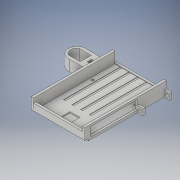
# Autodesk Inventor part: PI_Box_FINAL_COPY2
Saved by Autodesk Inventor 2017 (Build 210142000, 142)
## iProperties
Created: 2020-02-08
Part Number: PI_Box_FINAL_COPY2
Material: Generic
Document SubType Name: Modeling
Designer: S346559073
Density: 1 g/cm^3
Appearance: Default
Author: S346559073
Autodesk Inventor part; units mm, degrees
ref_plane "YZ Plane" through (0, 0, 0) normal (1, 0, 0) x (0, 1, 0)
ref_plane "XZ Plane" through (0, 0, 0) normal (0, 1, 0) x (-1, 0, 0)
ref_plane "XY Plane" through (0, 0, 0) normal (0, 0, 1) x (1, 0, 0)
sketch "Sketch1" plane through (0, 0, 0) normal (0, 1, 0) x (-1, 0, 0)
  line L0 (0, 0) -> (55.88, 0)
  line L1 (55.88, 0) -> (55.88, 88.9)
  line L2 (55.88, 88.9) -> (0, 88.9)
  line L3 (0, 88.9) -> (0, 0)
  dimension "d0" = 55.88
  dimension "d1" = 88.9
  constraints: 8 end point, 2 parallel, 1 horizontal, 1 perpendicular
  measures "d0" distance of L2.end L1.end
  measures "d1" distance of L0.end L1.end
extrude "Extrusion1" add sketch "Sketch1" along normal blind 2.54
sketch "Sketch2" plane through (0, 2.54, 0) normal (0, 1, 0) x (1, 0, 0)
  line L0 (-55.88, -88.9) -> (0, -88.9) projected
  line L1 (-22.86, -88.9) -> (-34.29, -88.9)
  line L2 (-34.29, -88.9) -> (-34.29, -72.771)
  line L3 (-34.29, -72.771) -> (-22.86, -72.771)
  line L4 (-22.86, -72.771) -> (-22.86, -88.9)
  point P0 (0, 0)
  dimension "d4" = 11.43
  dimension "d5" = 16.129
  dimension "d6" = 21.59
  dimension "d7" = 22.86
  constraints: 8 end point, 2 parallel, 1 horizontal, 1 perpendicular, 1 point on line
  measures "d4" distance of L2.end L3.end
  measures "d5" distance of L1.end L2.end
  measures "d6" distance of L0.start L1.end
  measures "d7" distance of L0.end L1.start
extrude "Extrusion2" cut sketch "Sketch2" against normal blind 1.27
sketch "Sketch3" plane through (0, 2.54, 0) normal (0, 1, 0) x (1, 0, 0)
  line L0 (-10.5239, -64.7488) -> (-8.3034, -64.7488)
  line L1 (-8.3034, -64.7488) -> (-8.3034, 0)
  line L2 (-8.3034, 0) -> (-10.5239, 0)
  line L3 (-10.5239, 0) -> (-10.5239, -64.7488)
  line L4 (0, 0) -> (-55.88, 0) projected
  line L5 (-27.9843, -64.7488) -> (-30.2048, -64.7488)
  line L6 (-30.2048, -64.7488) -> (-30.2048, 0)
  line L7 (-30.2048, 0) -> (-27.9843, 0)
  line L8 (-27.9843, 0) -> (-27.9843, -64.7488)
  line L9 (-49.8857, -64.7488) -> (-47.6652, -64.7488)
  line L10 (-47.6652, -64.7488) -> (-47.6652, 0)
  line L11 (-47.6652, 0) -> (-49.8857, 0)
  line L12 (-49.8857, 0) -> (-49.8857, -64.7488)
  line L13 (-40.0452, -64.7488) -> (-37.8248, -64.7488)
  line L14 (-37.8248, -64.7488) -> (-37.8248, 0)
  line L15 (-37.8248, 0) -> (-40.0452, 0)
  line L16 (-40.0452, 0) -> (-40.0452, -64.7488)
  line L17 (-20.3643, -64.7488) -> (-18.1439, -64.7488)
  line L18 (-18.1439, -64.7488) -> (-18.1439, 0)
  line L19 (-18.1439, 0) -> (-20.3643, 0)
  line L20 (-20.3643, 0) -> (-20.3643, -64.7488)
  line L21 (-47.6652, -64.7488) -> (-40.0452, -64.7488)
  line L22 (-34.29, -72.771) -> (-22.86, -72.771) projected
  line L23 (-37.8248, -64.7488) -> (-30.2048, -64.7488)
  line L24 (-27.9843, -64.7488) -> (-20.3643, -64.7488)
  line L25 (-18.1439, -64.7488) -> (-10.5239, -64.7488)
  dimension "d10" = 7.62
  constraints: 48 end point, 11 parallel, 9 collinear, 8 point on line, 6 perpendicular, 5 horizontal
  measures "d10" distance of L5.start L17.start
extrude "Extrusion3" cut sketch "Sketch3" against normal blind 0.508 contours L3 L2 L1 L0 | L17 L20 L4 L18 | L5 L6 L4 L8 | L13 L16 L4 L14 | L9 L12 L4 L10
sketch "Sketch4" plane through (-55.88, 0, 0) normal (-1, 0, 0) x (0, 0, 1)
  line L0 (88.9, 0) -> (0, 0) projected
  line L1 (88.9, 0) -> (0, 0)
  line L2 (0, 0) -> (0, 2.54)
  line L3 (0, 2.54) -> (88.9, 2.54)
  line L4 (88.9, 2.54) -> (88.9, 0)
  constraints: 8 end point, 2 parallel, 1 horizontal, 1 perpendicular
extrude "Extrusion4" add sketch "Sketch4" along normal blind 2.54
sketch "Sketch5" plane through (0, 2.54, 0) normal (0, 1, 0) x (1, 0, 0)
  line L0 (0, -88.9) -> (-58.42, -88.9) projected
  line L1 (-49.8857, 0) -> (-58.42, 0) projected
  line L2 (-58.42, -88.9) -> (-55.88, -88.9)
  line L3 (-55.88, -88.9) -> (-55.88, 0)
  line L4 (-55.88, 0) -> (-58.42, 0)
  line L5 (-58.42, 0) -> (-58.42, -88.9)
  point P0 (0, 0)
  dimension "d15" = 2.54
  constraints: 8 end point, 2 parallel, 1 horizontal, 1 perpendicular, 1 point on line
  measures "d15" distance of L4.end L3.end
extrude "Extrusion5" add sketch "Sketch5" along normal blind 12.7
sketch "Sketch6" plane through (0, 0, 88.9) normal (1, 0, 0) x (0, 0, -1)
  line L0 (0, 2.54) -> (16.129, 2.54) projected
  line L1 (0, 0) -> (88.9, 0) projected
  line L2 (0, 2.54) -> (88.9, 2.54)
  line L3 (88.9, 2.54) -> (88.9, 0)
  line L4 (88.9, 0) -> (0, 0)
  line L5 (0, 0) -> (0, 2.54)
  constraints: 8 end point, 2 parallel, 1 horizontal, 1 perpendicular
extrude "Extrusion6" add sketch "Sketch6" along normal blind 2.54
sketch "Sketch7" plane through (0, 2.54, 0) normal (0, 1, 0) x (1, 0, 0)
  line L0 (2.54, 0) -> (2.54, -88.9) projected
  line L1 (2.54, -88.9) -> (0, -88.9)
  line L2 (0, -88.9) -> (0, 0)
  line L3 (0, 0) -> (2.54, 0)
  line L4 (2.54, 0) -> (2.54, -88.9)
  constraints: 8 end point, 2 parallel, 1 horizontal, 1 perpendicular
extrude "Extrusion7" add sketch "Sketch7" along normal blind 12.7
sketch "Sketch8" plane through (-34.29, 1.27, 88.9) normal (0, 0, 1) x (1, 0, 0)
  line L0 (-24.13, -1.27) -> (-24.13, 13.97) projected
  line L1 (-21.59, 1.27) -> (-21.59, 13.97) projected
  line L2 (-24.13, 13.97) -> (-21.59, 13.97)
  line L3 (-21.59, 13.97) -> (-21.59, 1.27)
  line L4 (-21.59, 1.27) -> (-24.13, 1.27)
  line L5 (-24.13, 1.27) -> (-24.13, 13.97)
  line L6 (-24.13, 1.27) -> (36.83, 1.27)
  line L7 (36.83, 1.27) -> (36.83, 3.0441)
  line L8 (36.83, 3.0441) -> (-24.13, 3.0441)
  line L9 (-24.13, 3.0441) -> (-24.13, 1.27)
  line L10 (36.83, -1.27) -> (36.83, 13.97) projected
  line L11 (34.29, 1.27) -> (36.83, 1.27)
  line L12 (36.83, 1.27) -> (36.83, 13.97)
  line L13 (36.83, 13.97) -> (34.29, 13.97)
  line L14 (34.29, 13.97) -> (34.29, 1.27)
  line L15 (13.9257, 1.27) -> (6.3057, 1.27) projected
  line L16 (11.43, 0) -> (0, 0) projected
  line L17 (11.3074, 1.27) -> (0, 1.27)
  line L18 (0, 1.27) -> (0, 0)
  line L19 (0, 0) -> (11.3074, 0)
  line L20 (11.3074, 0) -> (11.3074, 1.27)
  point P0 (34.29, -1.27)
  constraints: 32 end point, 8 parallel, 4 horizontal, 4 perpendicular, 2 point on line
extrude "Extrusion8" add sketch "Sketch8" along normal blind 3.81 contours L0 L8 L1 L4 | L0 L2 L1 L8 | L1 L8 L14 L6 | L14 L13 L10 L8 | L8 L7 L6 L14
sketch "Sketch9" plane through (0, 2.54, 0) normal (0, 1, 0) x (1, 0, 0)
  line L0 (0, -92.71) -> (-55.88, -92.71) projected
  line L1 (-55.8607, -92.71) -> (0, -92.71)
  line L2 (0, -92.71) -> (0, -90.17)
  line L3 (0, -90.17) -> (-55.8607, -90.17)
  line L4 (-55.8607, -90.17) -> (-55.8607, -92.71)
  point P0 (0, 0)
  point P1 (-58.42, -92.71)
  point P2 (2.54, -92.71)
  dimension "d24" = 2.54
  constraints: 8 end point, 2 parallel, 1 horizontal, 1 perpendicular, 1 point on line
  measures "d24" distance of L3.end L1.start
extrude "Extrusion9" add sketch "Sketch9" along normal blind 7.62
sketch "Sketch10" plane through (-20.3643, 2.54, 0) normal (0, 0, -1) x (-1, 0, 0)
  line L0 (-22.9043, 0) -> (-22.9043, 12.7) projected
  line L1 (38.0557, -2.54) -> (38.0557, 12.7) projected
  line L2 (-22.9043, -3.3059) -> (38.0557, -3.3059)
  line L3 (38.0557, -3.3059) -> (38.0557, -0.2509)
  line L4 (38.0557, -0.2509) -> (-22.9043, -0.2509)
  line L5 (-22.9043, -0.2509) -> (-22.9043, -3.3059)
  point P0 (-20.3643, -2.54)
  constraints: 8 end point, 2 parallel, 1 horizontal, 1 perpendicular, 1 point on line
extrude "Extrusion10" add sketch "Sketch10" along normal blind 2.54
sketch "Sketch11" plane through (-49.8857, 2.2891, 0) normal (0, 1, 0) x (1, 0, 0)
  line L0 (52.4257, 2.54) -> (-8.5343, 2.54) projected
  line L1 (-8.5343, 0) -> (52.4257, 0)
  line L2 (52.4257, 0) -> (52.4257, 2.54)
  line L3 (52.4257, 2.54) -> (-8.5343, 2.54)
  line L4 (-8.5343, 2.54) -> (-8.5343, 0)
  point P0 (49.8857, 0)
  constraints: 8 end point, 2 parallel, 1 horizontal, 1 perpendicular
extrude "Extrusion12" add sketch "Sketch11" along normal blind 0.762
sketch "Sketch13" plane through (2.54, 0, 88.9) normal (1, 0, 0) x (0, 0, -1)
  line L0 (6.1993, 10.8195) -> (74.4262, 10.8195)
  line L1 (74.4262, 10.8195) -> (74.4262, 2.6915)
  line L2 (74.4262, 2.6915) -> (6.1993, 2.6915)
  line L3 (6.1993, 2.6915) -> (6.1993, 10.8195)
  line L4 (0, 2.54) -> (-3.81, 2.54) projected
  line L5 (0, 2.54) -> (0, 4.3141) projected
  point P0 (88.9, 0)
  dimension "d35" = 8.128
  dimension "d37" = 6.1993
  constraints: 8 end point, 2 parallel, 1 horizontal, 1 perpendicular
  measures "d35" distance of L0.end L1.end
  measures "d37" distance between parallel lines of L3 L5
extrude "Extrusion13" cut sketch "Sketch13" against normal blind 2.54
sketch "Sketch19" plane through (2.54, 2.6915, 82.7007) normal (0, 1, 0) x (1, 0, 0)
  line L0 (-2.54, -6.1993) -> (-2.54, 82.7007) projected
  line L1 (0, 68.2269) -> (0, 0) projected
  line L2 (-2.54, 68.7335) -> (0, 68.7335)
  line L3 (0, 68.7335) -> (0, 53.3001)
  line L4 (0, 53.3001) -> (-2.54, 53.3001)
  line L5 (-2.54, 53.3001) -> (-2.54, 68.7335)
  constraints: 8 end point, 2 parallel, 2 point on line, 1 horizontal, 1 perpendicular
extrude "Extrusion19" add sketch "Sketch19" along normal blind 10.16
sketch "Sketch20" plane through (2.54, 0, 88.9) normal (1, 0, 0) x (0, 0, -1)
  line L0 (56.0605, 2.54) -> (58.6005, 2.54)
  line L1 (58.6005, 2.54) -> (58.6005, 0)
  line L2 (58.6005, 0) -> (56.0605, 0)
  line L3 (56.0605, 0) -> (56.0605, 2.54)
  line L4 (88.9, 0) -> (0, 0) projected
  line L5 (89.1059, 2.54) -> (86.5659, 2.54)
  line L6 (86.5659, 2.54) -> (86.5659, 0)
  line L7 (86.5659, 0) -> (89.1059, 0)
  line L8 (89.1059, 0) -> (89.1059, 2.54)
  line L9 (0, 2.54) -> (88.9, 2.54) projected
  point P0 (57.3305, 0)
  dimension "d61" = 2.54
  dimension "d69" = 27.9654
  constraints: 16 end point, 4 parallel, 3 point on line, 2 horizontal, 2 perpendicular, 1 collinear, 1 horizontal alignment, 1 midpoint
  measures "d61" distance of L0.start L0.end
  measures "d69" distance of L6.end L1.end
extrude "Extrusion20" add sketch "Sketch20" along normal blind 5.08 contours L0 L1 L2 L3 | L5 L8 L7 L4 L6
sketch "Sketch21" plane through (2.54, 2.54, 32.8395) normal (0, 1, 0) x (1, 0, 0)
  line L0 (0, 2.54) -> (5.08, 2.54) projected
  line L1 (0, 0) -> (5.08, 0)
  line L2 (5.08, 0) -> (5.08, 2.54)
  line L3 (5.08, 2.54) -> (0, 2.54)
  line L4 (0, 2.54) -> (0, 0)
  line L5 (0, 33.0454) -> (5.08, 33.0454) projected
  line L6 (0, 30.5054) -> (5.08, 30.5054)
  line L7 (5.08, 30.5054) -> (5.08, 33.0454)
  line L8 (5.08, 33.0454) -> (0, 33.0454)
  line L9 (0, 33.0454) -> (0, 30.5054)
  point P0 (-2.54, 32.8395)
  constraints: 16 end point, 4 parallel, 2 horizontal, 2 perpendicular
extrude "Extrusion21" add sketch "Sketch21" along normal blind 2.54
sketch "Sketch23" plane through (-58.42, 0, 0) normal (-1, 0, 0) x (0, 0, 1)
  line L0 (17.272, 10.668) -> (25.908, 10.668)
  line L1 (25.908, 10.668) -> (25.908, 2.032)
  line L2 (25.908, 2.032) -> (17.272, 2.032)
  line L3 (17.272, 2.032) -> (17.272, 10.668)
  line L4 (0, 3.0511) -> (0, 15.24) projected
  line L5 (15.24, 12.7) -> (27.94, 12.7)
  line L6 (27.94, 12.7) -> (27.94, 0)
  line L7 (27.94, 0) -> (15.24, 0)
  line L8 (15.24, 0) -> (15.24, 12.7)
  line L9 (0, 0) -> (88.9, 0) projected
  dimension "d70" = 8.636
  dimension "d71" = 8.636
  dimension "d73" = 2.032
  dimension "d74" = 12.7
  dimension "d75" = 12.7
  dimension "d76" = 2.032
  dimension "d77" = 15.24
  constraints: 16 end point, 4 parallel, 2 horizontal, 2 perpendicular, 1 point on line
  measures "d70" distance of L0.end L1.end
  measures "d71" distance between parallel lines of L1 L3
  measures "d73" distance between parallel lines of L5 L0
  measures "d74" distance between parallel lines of L8 L6
  measures "d75" distance between parallel lines of L7 L5
  measures "d76" distance between parallel lines of L6 L1
  measures "d77" distance between parallel lines of L4 L8
extrude "Extrusion23" add sketch "Sketch23" along normal blind 9.144
sketch "Sketch24" plane through (-58.42, 12.7, 27.94) normal (0, 1, 0) x (1, 0, 0)
  arc A0 (-17.1656, 16.129) -> (-17.9509, -3.429) centre (-18.9636, 6.4064) ccw
  arc A1 (-23.114, 12.7) -> (-22.9376, 0) centre (-18.9636, 6.4064) ccw
  line L0 (0, 12.7) -> (-9.144, 12.7) projected
  line L1 (0, -3.429) -> (-17.9509, -3.429)
  line L2 (0, 16.129) -> (-17.1656, 16.129)
  line L3 (0, 12.7) -> (0, 16.129)
  line L4 (0, 0) -> (0, -3.429)
  line L5 (0, 0) -> (0, -3.429)
  line L6 (-9.144, 12.7) -> (-23.114, 12.7)
  line L7 (-9.144, 0) -> (-22.9376, 0)
  line L8 (0, 0) -> (-9.144, 0) projected
  line L9 (-9.144, 0) -> (0, 0)
  line L10 (0, 12.7) -> (-9.144, 12.7) projected
  line L11 (-9.144, 12.7) -> (0, 12.7)
  point P0 (58.42, 27.94)
  point P1 (-9.144, 1.0206)
  dimension "d101" = 3.429
  dimension "d104" = 3.429
  dimension "d105" = 13.97
  constraints: 18 end point, 4 horizontal, 4 point on circle, 2 centre point, 2 coincident, 1 collinear, 1 vertical
  measures "d101" distance of L0.start L2.start
  measures "d104" distance of L4.start L1.start
  measures "d105" distance of L0.end L6.end
sketch "Sketch25" plane through (-58.42, 12.7, 27.94) normal (0, 1, 0) x (1, 0, 0)
  line L0 (0, 27.94) -> (0, -64.77) projected
  line L1 (0, 3.81) -> (-5.08, 3.81)
  line L2 (-5.08, 3.81) -> (-5.08, 8.89)
  line L3 (-5.08, 8.89) -> (0, 8.89)
  line L4 (0, 8.89) -> (0, 3.81)
  line L5 (0, 0) -> (-9.144, 0) projected
  line L6 (0, 12.7) -> (-9.144, 12.7) projected
  point P0 (58.42, 27.94)
  point P1 (-18.1573, 0)
  point P2 (-18.1573, 12.7)
  point P3 (-22.9376, 0)
  point P4 (-23.114, 12.7)
  dimension "d84" = 5.08
  dimension "d85" = 5.08
  dimension "d87" = 3.81
  constraints: 8 end point, 2 parallel, 1 horizontal, 1 perpendicular, 1 point on line
  measures "d84" distance between parallel lines of L1 L3
  measures "d85" distance between parallel lines of L0 L2
  measures "d87" distance between parallel lines of L6 L3
extrude "Extrusion25" cut sketch "Sketch25" against normal blind 5.08
sketch "Sketch27" plane through (-58.42, -0.7659, 0) normal (0, -1, 0) x (1, 0, 0)
  line L0 (60.96, -2.54) -> (0, -2.54) projected
  line L1 (2.54, 0) -> (0, 0) projected
  line L2 (60.96, -2.54) -> (0, -2.54)
  line L3 (0, -2.54) -> (0, 0)
  line L4 (0, 0) -> (60.96, 0)
  line L5 (60.96, 0) -> (60.96, -2.54)
  point P0 (58.42, 0)
  constraints: 8 end point, 2 parallel, 1 horizontal, 1 perpendicular
extrude "Extrusion27" cut sketch "Sketch27" against normal blind 0.7645
sketch "Sketch28" plane through (2.54, 5.08, 32.8395) normal (0, 1, 0) x (1, 0, 0)
  line L0 (0, 2.54) -> (0, 0) projected
  line L1 (5.08, 0) -> (5.08, 2.54) projected
  line L2 (0, 2.54) -> (5.08, 2.54)
  line L3 (5.08, 2.54) -> (5.08, 0)
  line L4 (5.08, 0) -> (0, 0)
  line L5 (0, 0) -> (0, 2.54)
  line L6 (0, 33.0454) -> (0, 35.3795) projected
  line L7 (0, 30.5054) -> (5.08, 30.5054) projected
  line L8 (0, 33.0454) -> (5.08, 33.0454)
  line L9 (5.08, 33.0454) -> (5.08, 30.5054)
  line L10 (5.08, 30.5054) -> (0, 30.5054)
  line L11 (0, 30.5054) -> (0, 33.0454)
  point P0 (-2.54, 32.8395)
  constraints: 16 end point, 4 parallel, 2 horizontal, 2 perpendicular
extrude "Extrusion28" add sketch "Sketch28" along normal blind 1.905
sketch "Sketch29" plane through (7.62, 0, 88.9) normal (1, 0, 0) x (0, 0, -1)
  line L0 (56.0605, 2.6915) -> (56.0605, 6.985) projected
  line L1 (58.6005, 0) -> (58.6005, 6.985) projected
  line L2 (56.0605, 6.985) -> (58.6005, 6.985)
  line L3 (58.6005, 6.985) -> (58.6005, 0)
  line L4 (58.6005, 0) -> (56.0605, 0)
  line L5 (56.0605, 0) -> (56.0605, 6.985)
  line L6 (86.5659, 0) -> (86.5659, 6.985) projected
  line L7 (89.1059, 0) -> (89.1059, 6.985) projected
  line L8 (86.5659, 6.985) -> (89.1059, 6.985)
  line L9 (89.1059, 6.985) -> (89.1059, 0)
  line L10 (89.1059, 0) -> (86.5659, 0)
  line L11 (86.5659, 0) -> (86.5659, 6.985)
  point P0 (88.9, 0)
  constraints: 16 end point, 4 parallel, 2 horizontal, 2 perpendicular
extrude "Extrusion29" add sketch "Sketch29" along normal blind 1.27
sketch "Sketch30" plane through (0, 2.6915, 82.7007) normal (0, 1, 0) x (1, 0, 0)
  line L0 (2.54, 49.8612) -> (2.54, 0) projected
  line L1 (0, 53.3465) -> (2.54, 53.3465)
  line L2 (2.54, 53.3465) -> (2.54, 49.8612)
  line L3 (2.54, 49.8612) -> (0, 49.8612)
  line L4 (0, 49.8612) -> (0, 53.3465)
  point P0 (0, 82.7007)
  constraints: 8 end point, 2 parallel, 1 horizontal, 1 perpendicular
extrude "Extrusion30" add sketch "Sketch30" along normal blind 10.16
extrude "Extrusion31" add sketch "Sketch24" against normal blind 12.7
sketch "Sketch31" plane through (2.54, 0, -0.2059) normal (0, 0, -1) x (-1, 0, 0)
  circle A0 centre (-3.175, 3.4925) radius 1.905
  line L0 (0, 6.985) -> (-6.35, 6.985) projected
  line L1 (-6.35, 0) -> (-6.35, 6.985) projected
  point P0 (2.54, 0)
  point P1 (-3.175, 6.985)
  point P2 (-6.35, 3.4925)
  dimension "d108" = 3.81
  constraints: 2 midpoint, 1 centre point, 1 horizontal alignment, 1 vertical alignment
  measures "d108" diameter of A0
extrude "Extrusion32" cut sketch "Sketch31" against normal blind 35.56
sketch "Sketch36" plane through (2.54, 0, 88.9) normal (1, 0, 0) x (0, 0, -1)
  line L0 (6.1993, 10.8195) -> (6.1993, 2.6915) projected
  line L1 (6.1993, 2.6915) -> (2.9426, 2.6915)
  line L2 (2.9426, 2.6915) -> (2.9426, 10.8195)
  line L3 (2.9426, 10.8195) -> (6.1993, 10.8195)
  line L4 (6.1993, 10.8195) -> (6.1993, 2.6915)
  point P0 (88.9, 0)
  constraints: 8 end point, 2 parallel, 1 horizontal, 1 perpendicular
extrude "Extrusion34" cut sketch "Sketch36" against normal blind 3.175
sketch "Sketch37" plane through (0, 2.54, 0) normal (0, 1, 0) x (1, 0, 0)
  circle A0 centre (-3.5, -28.67) radius 1.375 projected
  circle A1 centre (-52.5, -28.67) radius 1.375 projected
  circle A2 centre (-52.5, -86.67) radius 1.375 projected
  circle A3 centre (-3.5, -86.67) radius 1.375 projected
  point P0 (0, 0)
extrude "Extrusion36" cut sketch "Sketch37" against normal blind 22.225
sketch "Sketch38" plane through (2.54, 0, 88.9) normal (1, 0, 0) x (0, 0, -1)
  line L0 (56.0605, 10.8195) -> (2.9426, 10.8195)
  line L1 (2.9426, 10.8195) -> (2.9426, 13.0489)
  line L2 (2.9426, 13.0489) -> (56.0605, 13.0489)
  line L3 (56.0605, 13.0489) -> (56.0605, 10.8195)
  point P0 (88.9, 0)
  constraints: 8 end point, 2 parallel, 1 horizontal, 1 perpendicular
extrude "Extrusion37" cut sketch "Sketch38" against normal blind 7.9375
body "Solid1"
